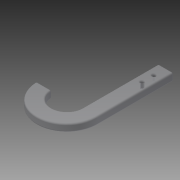
# Autodesk Inventor part: hook
Saved by Autodesk Inventor 2014 SP1 (Build 180222100, 222)
## iProperties
Created: 2013-12-24
Part Number: hook
Material: Polycarbonate, Clear
Document SubType Name: Modeling
Designer: RyanHughes
Density: 1.2 g/cm^3
Appearance: Polycarbonate - Clear
Author: RyanHughes
Autodesk Inventor part; units mm, degrees
ref_plane "YZ Plane" through (0, 0, 0) normal (1, 0, 0) x (0, 1, 0)
ref_plane "XZ Plane" through (0, 0, 0) normal (0, 1, 0) x (-1, 0, 0)
ref_plane "XY Plane" through (0, 0, 0) normal (0, 0, 1) x (1, 0, 0)
sketch "Sketch1" plane through (0, 0, 0) normal (0, 1, 0) x (-1, 0, 0)
  line L0 (-17.0496, -65.5906) -> (8.3504, -65.5906)
  line L1 (8.3504, -65.5906) -> (8.3504, 61.4094)
  line L2 (8.3504, 61.4094) -> (-17.0496, 61.4094)
  line L3 (-17.0496, 61.4094) -> (-17.0496, -65.5906)
  arc A0 (84.5504, 61.4094) -> (-17.0496, 61.4094) centre (33.7504, 61.4094) ccw
  arc A1 (59.1504, 61.4094) -> (8.3504, 61.4094) centre (33.7504, 61.4094) ccw
  line L4 (59.1504, 61.4094) -> (84.5504, 61.4094)
  point P0 (0, 0)
  dimension "d0" = 25.4
  dimension "d1" = 127
  dimension "d4" = 25.4
  constraints: 10 end point, 4 point on circle, 2 centre point, 2 parallel, 1 coincident, 1 collinear, 1 horizontal, 1 perpendicular, 1 tangent
  measures "d0" distance of L0.start L0.end
  measures "d1" distance of L0.end L1.end
  measures "d4" radius of A1
extrude "Extrusion1" add sketch "Sketch1" along normal blind 12.7
sketch "Sketch2" plane through (0, 12.7, 0) normal (0, 1, 0) x (1, 0, 0)
  line L0 (17.0496, -61.4094) -> (17.0496, 65.5906) projected
  line L1 (-8.3504, 65.5906) -> (-8.3504, -61.4094) projected
  circle A0 centre (4.3496, 45.3235) radius 2.2225
  circle A1 centre (4.3496, 25.8832) radius 2.2225
  line L2 (17.0496, 65.5906) -> (-8.3504, 0) construction
  line L3 (-8.3504, 65.5906) -> (17.0496, 0) construction
  line L4 (4.3496, 64.9234) -> (4.3496, 23.5933) construction
  point P0 (0, 0)
  point P1 (4.3496, 32.7953)
  dimension "d6" = 4.445
  dimension "d9" = 19.4403
  constraints: 6 end point, 4 point on line, 2 centre point, 1 midpoint, 1 parallel, 1 vertical, 2 other
  measures "d6" diameter of A0
  measures "d9" distance of A0.centre A1.centre
extrude "Extrusion2" cut sketch "Sketch2" against normal through all
fillet "Fillet2" radius 2.54 20 edges at (-33.7504, 0, 86.8094) (-8.3504, 0, -2.0906) (4.3496, 0, -65.5906) (17.0496, 0, -2.0906) (-33.7504, 0, 112.2094) (-71.8504, 0, 61.4094) (17.0496, 6.35, -65.5906) (17.0496, 12.7, -2.0906) (-8.3504, 12.7, -2.0906) (-8.3504, 6.35, -65.5906) (4.3496, 12.7, -65.5906) (-33.7504, 12.7, 112.2094) (-84.5504, 6.35, 61.4094) (-71.8504, 12.7, 61.4094) (-59.1504, 6.35, 61.4094) (-33.7504, 12.7, 86.8094) (2.1271, 12.7, -25.8832) (2.1271, 0, -25.8832) (2.1271, 12.7, -45.3235) (2.1271, 0, -45.3235)
body "Solid1"
